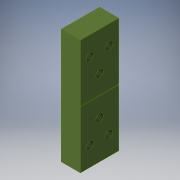
# Autodesk Inventor part: CabinetBraket
Saved by Autodesk Inventor 2019 (Build 230136000, 136)
## iProperties
Created: 2020-05-06
Part Number: CabinetBraket
Material: Generic
Document SubType Name: Modeling
Designer: james
Density: 1 g/cm^3
Appearance: Default(1)
Author: james
Autodesk Inventor part; units mm, degrees
ref_plane "YZ Plane" through (0, 0, 0) normal (1, 0, 0) x (0, 1, 0)
ref_plane "XZ Plane" through (0, 0, 0) normal (0, 1, 0) x (-1, 0, 0)
ref_plane "XY Plane" through (0, 0, 0) normal (0, 0, 1) x (1, 0, 0)
sketch "Sketch1" plane through (0, 0, 0) normal (1, 0, 0) x (0, 1, 0)
  line L0 (35.5795, 41.0894) -> (-40.6205, 41.0894)
  line L1 (-40.6205, 41.0894) -> (-40.6205, 15.6894)
  line L2 (-40.6205, 15.6894) -> (35.5795, 15.6894)
  line L3 (35.5795, 15.6894) -> (35.5795, 41.0894)
  point P0 (0, 0)
  dimension "d0" = 76.2
  dimension "d1" = 25.4
  constraints: 8 end point, 2 parallel, 1 horizontal, 1 perpendicular
  measures "d0" distance of L0.start L0.end
  measures "d1" distance of L2.end L0.start
extrude "Extrusion1" add sketch "Sketch1" along normal blind 12.7
sketch "Sketch2" plane through (12.7, 0, 0) normal (1, 0, 0) x (0, 0, -1)
  line L0 (-15.6894, -40.6205) -> (-15.6894, 35.5795) projected
  line L1 (-41.0894, 35.5795) -> (-41.0894, -40.6205) projected
  line L2 (-15.6894, 35.5795) -> (-41.0894, 35.5795) projected
  line L3 (-41.0894, -40.6205) -> (-15.6894, -40.6205) projected
  point P0 (0, 0)
  point P1 (-34.7394, 22.8795)
  point P2 (-22.0394, 22.8795)
  point P3 (-34.7394, -27.9205)
  point P4 (-22.0394, -27.9205)
  point P5 (-28.3894, -15.2205)
  point P6 (-28.3894, 10.1795)
  dimension "d4" = 0
  dimension "d5" = 0
  dimension "d6" = 6.35
  dimension "d7" = 6.35
  dimension "d8" = 12.7
  dimension "d9" = 25.4
  dimension "d10" = 12.7
  dimension "d11" = 25.4
  dimension "d12" = 12.7
  dimension "d13" = 6.35
  dimension "d14" = 6.35
  dimension "d15" = 12.7
  measures "d4" vertical distance of point (-22.039, 22.88) point (-34.739, 22.88)
  measures "d5" vertical distance of point (-22.039, -27.92) point (-34.739, -27.92)
  measures "d6" distance from line of L0 point (-22.039, 22.88)
  measures "d7" distance from line of L1 point (-34.739, 22.88)
  measures "d8" distance from line of L2 point (-34.739, 22.88)
  measures "d9" distance from line of L2 point (-28.389, 10.18)
  measures "d10" distance from line of L0 point (-28.389, 10.18)
  measures "d11" distance from line of L3 point (-28.389, -15.22)
  measures "d12" distance from line of L1 point (-28.389, -15.22)
  measures "d13" distance from line of L1 point (-34.739, -27.92)
  measures "d14" distance from line of L0 point (-22.039, -27.92)
  measures "d15" distance from line of L3 point (-22.039, -27.92)
hole "Hole1" at (12.7, 22.8795, 34.7394) at (12.7, 22.8795, 22.0394) at (12.7, -27.9205, 34.7394) at (12.7, -27.9205, 22.0394) at (12.7, -15.2205, 28.3894) at (12.7, 10.1795, 28.3894) direction (-1, 0, 0) diameter 4.9276 end through all
sketch "Sketch3" plane through (0, -40.6205, 41.0894) normal (0, 0, 1) x (1, 0, 0)
  arc A0 (12.7, 38.354) -> (12.7, 37.846) centre (12.7, 38.1) ccw
  line L0 (12.7, 76.2) -> (12.7, 0) projected
  line L1 (0, 76.2) -> (12.7, 76.2) projected
  point P0 (0, 40.6205)
  dimension "d23" = 0.254
  dimension "d24" = 38.1
  dimension "d27" = 0
  constraints: 2 point on circle, 2 point on line, 1 centre point
  measures "d23" radius of A0
  measures "d24" distance from line of A0.centre L1
  measures "d27" distance from line of L0 A0.centre
extrude "Extrusion2" cut sketch "Sketch3" against normal blind 26.9875
body "Solid1"
